Autodesk Inventor part; units mm, degrees
(part 3 of 3)
sketch "Эскиз6" plane through (0, 2, 0) normal (0, 1, 0) x (1, 0, 0)
  circle A0 centre (0, -40) radius 1.6 construction
  circle A1 centre (-46, 0) radius 1.6 construction
  circle A2 centre (46, 0) radius 1.6 construction
  line L0 (-6.2595, 46.1335) -> (-19.2746, 46.1335) construction
  arc A3 (-19.2746, 46.1335) -> (-21.6698, 47.1257) centre (-21.9203, 43.1335) ccw construction
  line L1 (-21.6698, 47.1257) -> (-42.4264, 67.8823) construction
  line L2 (-42.4264, 67.8823) -> (-34.2947, 76.014) construction
  arc A4 (-34.2947, 76.014) -> (-34.2947, 83.085) centre (-37.8302, 79.5495) ccw construction
  line L3 (-34.2947, 83.085) -> (-38.3892, 87.1795) construction
  arc A5 (-37.7453, 90.4395) -> (-38.3892, 87.1795) centre (-36.975, 88.5938) ccw construction
  arc A6 (-25.8102, 94.5401) -> (-37.7453, 90.4395) centre (0, 0) ccw construction
  arc A7 (-25.8102, 94.5401) -> (-20.7476, 95.7786) centre (-24, 98.1071) ccw construction
  arc A8 (20.7476, 95.7786) -> (-20.7476, 95.7786) centre (0, 0) ccw construction
  arc A9 (20.7476, 95.7786) -> (25.8102, 94.5401) centre (24, 98.1071) ccw construction
  arc A10 (37.7453, 90.4395) -> (25.8102, 94.5401) centre (0, 0) ccw construction
  arc A11 (38.3892, 87.1795) -> (37.7453, 90.4395) centre (36.975, 88.5938) ccw construction
  line L4 (38.3892, 87.1795) -> (34.2947, 83.085) construction
  arc A12 (34.2947, 83.085) -> (34.2947, 76.014) centre (37.8302, 79.5495) ccw construction
  line L5 (34.2947, 76.014) -> (42.4264, 67.8823) construction
  line L6 (42.4264, 67.8823) -> (21.6698, 47.1257) construction
  arc A13 (21.6698, 47.1257) -> (19.2746, 46.1335) centre (21.9203, 43.1335) ccw construction
  line L7 (19.2746, 46.1335) -> (6.2595, 46.1335) construction
  arc A14 (3.5768, 47.7906) -> (6.2595, 46.1335) centre (6.2595, 49.1335) ccw construction
  arc A15 (3.5768, 47.7906) -> (-3.5768, 47.7906) centre (0, 46) ccw construction
  arc A16 (-6.2595, 46.1335) -> (-3.5768, 47.7906) centre (-6.2595, 49.1335) ccw construction
  arc A17 (48.6481, 93.0503) -> (-48.6481, 93.0503) centre (0, 0) ccw construction
  arc A18 (-48.6481, 93.0503) -> (-49.3795, 88.2704) centre (-47.2582, 90.3917) ccw construction
  line L8 (-49.3795, 88.2704) -> (-46.3155, 85.2064) construction
  arc A19 (-46.3155, 73.8927) -> (-46.3155, 85.2064) centre (-51.9723, 79.5495) ccw construction
  line L9 (-46.3155, 73.8927) -> (-73.8927, 46.3155) construction
  arc A20 (-85.2064, 46.3155) -> (-73.8927, 46.3155) centre (-79.5495, 51.9723) ccw construction
  line L10 (-85.2064, 46.3155) -> (-88.2704, 49.3795) construction
  arc A21 (-88.2704, 49.3795) -> (-93.0503, 48.6481) centre (-90.3917, 47.2582) ccw construction
  arc A22 (-93.0503, 48.6481) -> (-93.0503, -48.6481) centre (0, 0) ccw construction
  arc A23 (-93.0503, -48.6481) -> (-88.2704, -49.3795) centre (-90.3917, -47.2582) ccw construction
  line L11 (-88.2704, -49.3795) -> (-85.2064, -46.3155) construction
  arc A24 (-73.8927, -46.3155) -> (-85.2064, -46.3155) centre (-79.5495, -51.9723) ccw construction
  line L12 (-73.8927, -46.3155) -> (-46.3155, -73.8927) construction
  arc A25 (-46.3155, -85.2064) -> (-46.3155, -73.8927) centre (-51.9723, -79.5495) ccw construction
  line L13 (-46.3155, -85.2064) -> (-49.3795, -88.2704) construction
  arc A26 (-49.3795, -88.2704) -> (-48.6481, -93.0503) centre (-47.2582, -90.3917) ccw construction
  arc A27 (-48.6481, -93.0503) -> (-45.42, -94.668) centre (0, 0) ccw construction
  arc A28 (-45.42, -94.668) -> (-43.0355, -94.1655) centre (-44.5548, -92.8648) ccw construction
  line L14 (-43.0355, -94.1655) -> (-18.3802, -65.3664) construction
  arc A29 (-17.477, -64.7643) -> (-18.3802, -65.3664) centre (-16.8609, -66.6671) ccw construction
  line L15 (-17.477, -64.7643) -> (-0.6161, -59.3045) construction
  arc A30 (0.6161, -59.3045) -> (-0.6161, -59.3045) centre (0, -61.2072) ccw construction
  line L16 (0.6161, -59.3045) -> (17.477, -64.7643) construction
  arc A31 (18.3802, -65.3664) -> (17.477, -64.7643) centre (16.8609, -66.6671) ccw construction
  line L17 (18.3802, -65.3664) -> (43.0355, -94.1655) construction
  arc A32 (43.0355, -94.1655) -> (45.42, -94.668) centre (44.5548, -92.8648) ccw construction
  arc A33 (45.42, -94.668) -> (48.6481, -93.0503) centre (0, 0) ccw construction
  arc A34 (48.6481, -93.0503) -> (49.3795, -88.2704) centre (47.2582, -90.3917) ccw construction
  line L18 (49.3795, -88.2704) -> (46.3155, -85.2064) construction
  arc A35 (46.3155, -73.8927) -> (46.3155, -85.2064) centre (51.9723, -79.5495) ccw construction
  line L19 (46.3155, -73.8927) -> (73.8927, -46.3155) construction
  arc A36 (85.2064, -46.3155) -> (73.8927, -46.3155) centre (79.5495, -51.9723) ccw construction
  line L20 (85.2064, -46.3155) -> (88.2704, -49.3795) construction
  arc A37 (88.2704, -49.3795) -> (93.0503, -48.6481) centre (90.3917, -47.2582) ccw construction
  arc A38 (93.0503, -48.6481) -> (93.0503, 48.6481) centre (0, 0) ccw construction
  arc A39 (93.0503, 48.6481) -> (88.2704, 49.3795) centre (90.3917, 47.2582) ccw construction
  line L21 (88.2704, 49.3795) -> (85.2064, 46.3155) construction
  arc A40 (73.8927, 46.3155) -> (85.2064, 46.3155) centre (79.5495, 51.9723) ccw construction
  line L22 (73.8927, 46.3155) -> (46.3155, 73.8927) construction
  arc A41 (46.3155, 85.2064) -> (46.3155, 73.8927) centre (51.9723, 79.5495) ccw construction
  line L23 (46.3155, 85.2064) -> (49.3795, 88.2704) construction
  arc A42 (49.3795, 88.2704) -> (48.6481, 93.0503) centre (47.2582, 90.3917) ccw construction
  circle A43 centre (-24, 98.1071) radius 1.6 construction
  arc A44 (47.7906, -3.5768) -> (46.1335, -6.2595) centre (49.1335, -6.2595) ccw construction
  arc A45 (47.7906, -3.5768) -> (47.7906, 3.5768) centre (46, 0) ccw construction
  arc A46 (46.1335, 6.2595) -> (47.7906, 3.5768) centre (49.1335, 6.2595) ccw construction
  line L24 (46.1335, 6.2595) -> (46.1335, 19.2746) construction
  arc A47 (46.1335, 19.2746) -> (47.1257, 21.6698) centre (43.1335, 21.9203) ccw construction
  line L25 (47.1257, 21.6698) -> (67.8823, 42.4264) construction
  line L26 (67.8823, 42.4264) -> (76.014, 34.2947) construction
  arc A48 (76.014, 34.2947) -> (83.085, 34.2947) centre (79.5495, 37.8302) ccw construction
  line L27 (83.085, 34.2947) -> (87.1795, 38.3892) construction
  arc A49 (90.4395, 37.7453) -> (87.1795, 38.3892) centre (88.5938, 36.975) ccw construction
  arc A50 (97.9653, 2.6059) -> (90.4395, 37.7453) centre (0, 0) ccw construction
  arc A51 (97.9653, 2.6059) -> (97.9653, -2.6059) centre (101, 0) ccw construction
  arc A52 (90.4395, -37.7453) -> (97.9653, -2.6059) centre (0, 0) ccw construction
  arc A53 (87.1795, -38.3892) -> (90.4395, -37.7453) centre (88.5938, -36.975) ccw construction
  line L28 (87.1795, -38.3892) -> (83.085, -34.2947) construction
  arc A54 (83.085, -34.2947) -> (76.014, -34.2947) centre (79.5495, -37.8302) ccw construction
  line L29 (76.014, -34.2947) -> (67.8823, -42.4264) construction
  line L30 (67.8823, -42.4264) -> (47.1257, -21.6698) construction
  arc A55 (47.1257, -21.6698) -> (46.1335, -19.2746) centre (43.1335, -21.9203) ccw construction
  line L31 (46.1335, -19.2746) -> (46.1335, -6.2595) construction
  circle A56 centre (101, 0) radius 1.6 construction
  circle A57 centre (-101, 0) radius 1.6 construction
  arc A58 (-47.7906, 3.5768) -> (-46.1335, 6.2595) centre (-49.1335, 6.2595) ccw construction
  arc A59 (-47.7906, 3.5768) -> (-47.7906, -3.5768) centre (-46, 0) ccw construction
  arc A60 (-46.1335, -6.2595) -> (-47.7906, -3.5768) centre (-49.1335, -6.2595) ccw construction
  line L32 (-46.1335, -6.2595) -> (-46.1335, -19.2746) construction
  arc A61 (-46.1335, -19.2746) -> (-47.1257, -21.6698) centre (-43.1335, -21.9203) ccw construction
  line L33 (-47.1257, -21.6698) -> (-67.8823, -42.4264) construction
  line L34 (-67.8823, -42.4264) -> (-76.014, -34.2947) construction
  arc A62 (-76.014, -34.2947) -> (-83.085, -34.2947) centre (-79.5495, -37.8302) ccw construction
  line L35 (-83.085, -34.2947) -> (-87.1795, -38.3892) construction
  arc A63 (-90.4395, -37.7453) -> (-87.1795, -38.3892) centre (-88.5938, -36.975) ccw construction
  arc A64 (-97.9653, -2.6059) -> (-90.4395, -37.7453) centre (0, 0) ccw construction
  arc A65 (-97.9653, -2.6059) -> (-97.9653, 2.6059) centre (-101, 0) ccw construction
  arc A66 (-90.4395, 37.7453) -> (-97.9653, 2.6059) centre (0, 0) ccw construction
  arc A67 (-87.1795, 38.3892) -> (-90.4395, 37.7453) centre (-88.5938, 36.975) ccw construction
  line L36 (-87.1795, 38.3892) -> (-83.085, 34.2947) construction
  arc A68 (-83.085, 34.2947) -> (-76.014, 34.2947) centre (-79.5495, 37.8302) ccw construction
  line L37 (-76.014, 34.2947) -> (-67.8823, 42.4264) construction
  line L38 (-67.8823, 42.4264) -> (-47.1257, 21.6698) construction
  arc A69 (-47.1257, 21.6698) -> (-46.1335, 19.2746) centre (-43.1335, 21.9203) ccw construction
  line L39 (-46.1335, 19.2746) -> (-46.1335, 6.2595) construction
  circle A70 centre (45.1111, -90.3659) radius 1.6 construction
  circle A71 centre (45.1111, 90.3659) radius 1.6 construction
  circle A72 centre (90.3659, 45.1111) radius 1.6 construction
  circle A73 centre (-45.1111, -90.3659) radius 1.6 construction
  circle A74 centre (90.3659, -45.1111) radius 1.6 construction
  circle A75 centre (-45.1111, 90.3659) radius 1.6 construction
  circle A76 centre (-90.3659, 45.1111) radius 1.6 construction
  circle A77 centre (-90.3659, -45.1111) radius 1.6 construction
  line L40 (63.6396, 46.669) -> (43.8406, 26.8701) construction
  arc A78 (41.0122, 26.8701) -> (43.8406, 26.8701) centre (42.4264, 28.2843) ccw construction
  line L41 (41.0122, 26.8701) -> (26.8701, 41.0122) construction
  arc A79 (26.8701, 43.8406) -> (26.8701, 41.0122) centre (28.2843, 42.4264) ccw construction
  line L42 (26.8701, 43.8406) -> (46.669, 63.6396) construction
  line L43 (46.669, 63.6396) -> (63.6396, 46.669) construction
  line L44 (-46.669, 63.6396) -> (-26.8701, 43.8406) construction
  arc A80 (-26.8701, 41.0122) -> (-26.8701, 43.8406) centre (-28.2843, 42.4264) ccw construction
  line L45 (-26.8701, 41.0122) -> (-41.0122, 26.8701) construction
  arc A81 (-43.8406, 26.8701) -> (-41.0122, 26.8701) centre (-42.4264, 28.2843) ccw construction
  line L46 (-43.8406, 26.8701) -> (-63.6396, 46.669) construction
  line L47 (-63.6396, 46.669) -> (-46.669, 63.6396) construction
  line L48 (-63.6396, -46.669) -> (-43.8406, -26.8701) construction
  arc A82 (-41.0122, -26.8701) -> (-43.8406, -26.8701) centre (-42.4264, -28.2843) ccw construction
  line L49 (-41.0122, -26.8701) -> (-26.8701, -41.0122) construction
  arc A83 (-26.8701, -43.8406) -> (-26.8701, -41.0122) centre (-28.2843, -42.4264) ccw construction
  line L50 (-26.8701, -43.8406) -> (-46.669, -63.6396) construction
  line L51 (-46.669, -63.6396) -> (-63.6396, -46.669) construction
  line L52 (-42.4264, -67.8823) -> (-21.6698, -47.1257) construction
  arc A84 (-21.6698, -47.1257) -> (-19.2746, -46.1335) centre (-21.9203, -43.1335) ccw construction
  line L53 (-19.2746, -46.1335) -> (19.2746, -46.1335) construction
  arc A85 (19.2746, -46.1335) -> (21.6698, -47.1257) centre (21.9203, -43.1335) ccw construction
  line L54 (21.6698, -47.1257) -> (42.4264, -67.8823) construction
  line L55 (42.4264, -67.8823) -> (37.1244, -73.1843) construction
  arc A86 (34.1909, -73.0707) -> (37.1244, -73.1843) centre (35.7102, -71.7701) ccw construction
  line L56 (34.1909, -73.0707) -> (25.4187, -62.8242) construction
  arc A87 (24.842, -61.8893) -> (25.4187, -62.8242) centre (28.1154, -60.5155) ccw construction
  line L57 (24.842, -61.8893) -> (23.8313, -59.4808) construction
  arc A88 (23.8313, -59.4808) -> (21.0049, -57.3328) centre (20.5578, -60.8546) ccw construction
  line L58 (21.0049, -57.3328) -> (15.1585, -56.5907) construction
  arc A89 (14.5119, -56.4463) -> (15.1585, -56.5907) centre (15.6055, -53.069) ccw construction
  line L59 (14.5119, -56.4463) -> (0.6161, -51.9466) construction
  arc A90 (0.6161, -51.9466) -> (-0.6161, -51.9466) centre (0, -53.8493) ccw construction
  line L60 (-0.6161, -51.9466) -> (-14.5119, -56.4463) construction
  arc A91 (-15.1585, -56.5907) -> (-14.5119, -56.4463) centre (-15.6055, -53.069) ccw construction
  line L61 (-15.1585, -56.5907) -> (-21.0049, -57.3328) construction
  arc A92 (-21.0049, -57.3328) -> (-23.8313, -59.4808) centre (-20.5578, -60.8546) ccw construction
  line L62 (-23.8313, -59.4808) -> (-24.842, -61.8893) construction
  arc A93 (-25.4187, -62.8242) -> (-24.842, -61.8893) centre (-28.1154, -60.5155) ccw construction
  line L63 (-25.4187, -62.8242) -> (-34.1909, -73.0707) construction
  arc A94 (-37.1244, -73.1843) -> (-34.1909, -73.0707) centre (-35.7102, -71.7701) ccw construction
  line L64 (-37.1244, -73.1843) -> (-42.4264, -67.8823) construction
  circle A95 centre (43.1335, 21.9203) radius 1.6 construction
  circle A96 centre (21.9203, -43.1335) radius 1.6 construction
  circle A97 centre (-21.9203, -43.1335) radius 1.6 construction
  circle A98 centre (-43.1335, -21.9203) radius 1.6 construction
  circle A99 centre (-43.1335, 21.9203) radius 1.6 construction
  circle A100 centre (-21.9203, 43.1335) radius 1.6 construction
  circle A101 centre (43.1335, -21.9203) radius 1.6 construction
  circle A102 centre (21.9203, 43.1335) radius 1.6 construction
  circle A103 centre (-37.8302, 79.5495) radius 1.6 construction
  circle A104 centre (-79.5495, 37.8302) radius 1.6 construction
  circle A105 centre (-79.5495, -37.8302) radius 1.6 construction
  circle A106 centre (79.5495, -37.8302) radius 1.6 construction
  circle A107 centre (37.8302, 79.5495) radius 1.6 construction
  circle A108 centre (79.5495, 37.8302) radius 1.6 construction
  circle A109 centre (-20.5578, -60.8546) radius 1.55 construction
  circle A110 centre (20.5578, -60.8546) radius 1.55 construction
  circle A111 centre (37.8302, -79.5495) radius 1.6 construction
  circle A112 centre (-37.8302, -79.5495) radius 1.6 construction
  line L65 (46.669, -63.6396) -> (26.8701, -43.8406) construction
  arc A113 (26.8701, -41.0122) -> (26.8701, -43.8406) centre (28.2843, -42.4264) ccw construction
  line L66 (26.8701, -41.0122) -> (41.0122, -26.8701) construction
  arc A114 (43.8406, -26.8701) -> (41.0122, -26.8701) centre (42.4264, -28.2843) ccw construction
  line L67 (43.8406, -26.8701) -> (63.6396, -46.669) construction
  line L68 (63.6396, -46.669) -> (46.669, -63.6396) construction
  circle A115 centre (24, 98.1071) radius 1.6 construction
  circle A116 centre (0, 46) radius 1.6 construction
  arc A117 (3.6492, -38.362) -> (6.3862, -40.1335) centre (6.3862, -37.1335) ccw construction
  arc A118 (3.6492, -38.362) -> (-3.6492, -38.362) centre (0, -40) ccw construction
  arc A119 (-6.3862, -40.1335) -> (-3.6492, -38.362) centre (-6.3862, -37.1335) ccw construction
  line L69 (-6.3862, -40.1335) -> (-19.2746, -40.1335) construction
  arc A120 (-19.2746, -40.1335) -> (-21.6698, -39.1414) centre (-21.9203, -43.1335) ccw construction
  line L70 (-21.6698, -39.1414) -> (-39.1414, -21.6698) construction
  arc A121 (-39.1414, -21.6698) -> (-40.1335, -19.2746) centre (-43.1335, -21.9203) ccw construction
  line L71 (-40.1335, -19.2746) -> (-40.1335, 19.2746) construction
  arc A122 (-40.1335, 19.2746) -> (-39.1414, 21.6698) centre (-43.1335, 21.9203) ccw construction
  line L72 (-39.1414, 21.6698) -> (-21.6698, 39.1414) construction
  arc A123 (-21.6698, 39.1414) -> (-19.2746, 40.1335) centre (-21.9203, 43.1335) ccw construction
  line L73 (-19.2746, 40.1335) -> (19.2746, 40.1335) construction
  arc A124 (19.2746, 40.1335) -> (21.6698, 39.1414) centre (21.9203, 43.1335) ccw construction
  line L74 (21.6698, 39.1414) -> (39.1414, 21.6698) construction
  arc A125 (39.1414, 21.6698) -> (40.1335, 19.2746) centre (43.1335, 21.9203) ccw construction
  line L75 (40.1335, 19.2746) -> (40.1335, -19.2746) construction
  arc A126 (40.1335, -19.2746) -> (39.1414, -21.6698) centre (43.1335, -21.9203) ccw construction
  line L76 (39.1414, -21.6698) -> (21.6698, -39.1414) construction
  arc A127 (21.6698, -39.1414) -> (19.2746, -40.1335) centre (21.9203, -43.1335) ccw construction
  line L77 (19.2746, -40.1335) -> (6.3862, -40.1335) construction
  line L78 (0, 0) -> (0, 105) construction
  arc A128 (48.6481, 93.0503) -> (-48.6481, 93.0503) centre (0, 0) ccw construction
  line L79 (-19.5, 5.5231) -> (19.5, 5.5231) construction
  line L80 (19.5, 5.5231) -> (19.5, 136.6901) construction
  line L81 (19.5, 136.6901) -> (-19.5, 136.6901) construction
  line L82 (-19.5, 136.6901) -> (-19.5, 5.5231) construction
  circle A129 centre (-24, 98.1071) radius 4 construction
  circle A130 centre (24, 98.1071) radius 4 construction
  arc A131 (-21.3158, 95.1414) -> (20.4598, 95.3292) centre (0, 0) ccw construction
  arc A132 (-23.5, 93.6349) -> (-20.4598, 95.3292) centre (-24, 98.1071) ccw
  line L83 (-23.5, 49.663) -> (-23.5, 93.6349)
  line L84 (-20, 47.2032) -> (-20, 95.4267)
  arc A133 (-19.0919, 46.6335) -> (-21.4454, 47.6084) centre (-21.9203, 43.1335) ccw
  line L85 (-21.4454, 47.6084) -> (-23.5, 49.663)
  line L86 (-21.6698, 47.1257) -> (-42.4264, 67.8823) construction
  line L87 (-42.4264, 67.8823) -> (-34.2947, 76.014) construction
  line L88 (-19.0919, 46.6335) -> (-6.5611, 46.6335)
  arc A134 (0, 41.5) -> (3.9366, 48.1801) centre (0, 46) ccw construction
  arc A135 (-4.4552, 46.6335) -> (0, 41.5) centre (0, 46) ccw construction
  arc A136 (-6.5611, 46.6335) -> (-3.9366, 48.1801) centre (-6.5611, 49.6335) ccw
  line L89 (-23.5, 49.663) -> (-42.0729, 68.2358) construction
  arc A137 (-18.5662, 46.1335) -> (-19.0919, 46.6335) centre (-21.9203, 43.1335) ccw construction
  arc A138 (-21.4454, 47.6084) -> (-18.5662, 46.1335) centre (-21.9203, 43.1335) ccw construction
  arc A139 (-25.858, 94.0086) -> (-23.5, 93.6349) centre (-24, 98.1071) ccw construction
  arc A140 (-20.4598, 95.3292) -> (-25.858, 94.0086) centre (-24, 98.1071) ccw construction
  arc A141 (-20.4598, 95.3292) -> (-21.3158, 95.1414) centre (0, 0) ccw construction
  arc A142 (20.4598, 95.3292) -> (23.5, 93.6349) centre (24, 98.1071) ccw
  line L90 (23.5, 49.663) -> (23.5, 93.6349)
  line L91 (20, 47.2032) -> (20, 95.4267)
  arc A143 (21.4454, 47.6084) -> (19.0919, 46.6335) centre (21.9203, 43.1335) ccw
  line L92 (21.4454, 47.6084) -> (23.5, 49.663)
  line L93 (19.0919, 46.6335) -> (6.5611, 46.6335)
  arc A144 (3.9366, 48.1801) -> (6.5611, 46.6335) centre (6.5611, 49.6335) ccw
  arc A145 (3.9366, 48.1801) -> (-3.9366, 48.1801) centre (0, 46) ccw
  arc A146 (20.4598, 95.3292) -> (-20.4598, 95.3292) centre (0, 0) ccw
  dimension "d26" = 360
  dimension "d112" = 8
  dimension "d111" = 39
  dimension "d113" = 0.5
  dimension "d114" = 9
  dimension "d115" = 4
  dimension "d116" = 0.5
  dimension "d117" = 9
  dimension "d118" = 0.5
  dimension "d119" = 0.5
  dimension "d120" = 9
  dimension "d121" = 3
  constraints: 42 point on circle, 28 end point, 17 centre point, 13 symmetric about line, 5 coincident, 4 parallel, 4 point on line, 2 horizontal, 2 tangent, 2 vertical, 1 perpendicular, 8 other
  measures "d111" distance of L81.end L80.end
  measures "d113" radial gap between concentric circles of A8 A131
  measures "d114" diameter of A132
  measures "d115" distance between parallel lines of L82 L83
  measures "d116" distance between parallel lines of L82 L84
  measures "d117" diameter of A133
  measures "d118" distance between parallel lines of L86 L85
  measures "d119" distance between parallel lines of L0 L88
  measures "d120" diameter of A134
  measures "d121" radius of A136
extrude "Выдавливание9" add sketch "Эскиз6" along normal blind 1.85 and the other way blind 2
extrude "Выдавливание10" add sketch "Эскиз6" along normal blind 7 contours A132 A146 L84 A133 L85 L83 | A146 A142 L90 L92 A143 L91
ref_plane "РабПлоскость1" through (0, 9, 0) normal (0, 1, 0) x (1, 0, 0)
sketch "Эскиз7" plane through (0, 9, 0) normal (0, 1, 0) x (1, 0, 0)
  line L0 (-20, 95.4267) -> (-20, 47.2032) projected
  arc A0 (-19.0919, 46.6335) -> (-20, 47.2032) centre (-21.9203, 43.1335) ccw projected
  line L1 (-19.0919, 46.6335) -> (-6.5611, 46.6335) projected
  arc A1 (-6.5611, 46.6335) -> (-3.9366, 48.1801) centre (-6.5611, 49.6335) ccw construction
  arc A2 (3.9366, 48.1801) -> (-3.9366, 48.1801) centre (0, 46) ccw construction
  arc A3 (3.9366, 48.1801) -> (6.5611, 46.6335) centre (6.5611, 49.6335) ccw construction
  line L2 (6.5611, 46.6335) -> (19.0919, 46.6335) projected
  arc A4 (20, 47.2032) -> (19.0919, 46.6335) centre (21.9203, 43.1335) ccw projected
  line L3 (20, 47.2032) -> (20, 95.4267) projected
  arc A5 (20, 95.4267) -> (-20, 95.4267) centre (0, 0) ccw projected
  arc A6 (-20, 95.4267) -> (-20.4598, 95.3292) centre (0, 0) ccw projected
  arc A7 (-23.5, 93.6349) -> (-20.4598, 95.3292) centre (-24, 98.1071) ccw projected
  line L4 (-23.5, 93.6349) -> (-23.5, 49.663) projected
  line L5 (-23.5, 49.663) -> (-21.4454, 47.6084) projected
  arc A8 (-20, 47.2032) -> (-21.4454, 47.6084) centre (-21.9203, 43.1335) ccw projected
  line L6 (-20, 47.2032) -> (-20, 95.4267) projected
  arc A9 (20.4598, 95.3292) -> (20, 95.4267) centre (0, 0) ccw projected
  line L7 (20, 95.4267) -> (20, 47.2032) projected
  arc A10 (21.4454, 47.6084) -> (20, 47.2032) centre (21.9203, 43.1335) ccw projected
  line L8 (21.4454, 47.6084) -> (23.5, 49.663) projected
  line L9 (23.5, 49.663) -> (23.5, 93.6349) projected
  arc A11 (20.4598, 95.3292) -> (23.5, 93.6349) centre (24, 98.1071) ccw projected
  line L10 (18.2, 46.6335) -> (18.2, 95.7863)
  arc A12 (3.5768, 47.7906) -> (-3.5768, 47.7906) centre (0, 46) ccw construction
  line L11 (0, 46) -> (0, 97.5) construction
  line L12 (-18.2, 46.6335) -> (-18.2, 95.7863)
  point P0 (-20, 95.4267)
  point P1 (20, 95.4267)
  dimension "d129" = 1.8
  constraints: 6 end point, 2 point on circle, 2 symmetric about line, 1 point on line, 1 vertical
  measures "d129" distance between parallel lines of L3 L10
extrude "Выдавливание11" add sketch "Эскиз7" along normal blind 5
chamfer "Фаска1" distance 1.8 angle 45 2 edges at (18.2, 9, -71.2099) (-18.2, 9, -71.2099)
fillet "Сопряжение1" radius 3 2 edges at (23.5, 14, -71.6489) (-23.5, 14, -71.6489)
fillet "Сопряжение2" radius 1 2 edges at (18.2, 14, -71.2099) (-18.2, 14, -71.2099)
ref_plane "РабПлоскость2" through (6.5611, 3.85, -46.6335) normal (0, 0, 1) x (1, 0, 0)
sketch "Эскиз8" plane through (6.5611, 3.85, -46.6335) normal (0, 0, 1) x (1, 0, 0)
  line L0 (-26.5611, 0) -> (-25.6529, 0) construction
  line L1 (-25.6529, 0) -> (-13.1221, 0) construction
  line L2 (-13.1221, 0) -> (-10.4977, 0) construction
  line L3 (-10.4977, 0) -> (-2.6244, 0) construction
  line L4 (-2.6244, 0) -> (0, 0) construction
  line L5 (0, 0) -> (12.5308, 0) construction
  line L6 (12.5308, 0) -> (13.4389, 0) construction
  line L7 (13.4389, 0) -> (-26.5611, 0) construction
  line L8 (-24.7611, 6.95) -> (-24.7611, 9.15) construction
  line L9 (-26.5611, 5.15) -> (-24.7611, 6.95) construction
  line L10 (-26.5611, 0) -> (-26.5611, 5.15) construction
  line L11 (13.4389, 0) -> (-26.5611, 0) construction
  line L12 (13.4389, 0) -> (13.4389, 5.15) construction
  line L13 (11.6389, 6.95) -> (13.4389, 5.15) construction
  line L14 (11.6389, 6.95) -> (11.6389, 9.15) construction
  line L15 (13.8987, 10.15) -> (12.6389, 10.15) construction
  line L16 (13.8987, -3.85) -> (13.8987, 10.15) construction
  line L17 (-27.0209, -3.85) -> (13.8987, -3.85) construction
  line L18 (-27.0209, -3.85) -> (-27.0209, 10.15) construction
  line L19 (-25.7611, 10.15) -> (-27.0209, 10.15) construction
  line L20 (-27.0209, 10.15) -> (-27.0611, 10.15) construction
  line L21 (-27.0209, -3.85) -> (-27.0209, 10.15) construction
  line L22 (-30.0611, -3.85) -> (-27.0209, -3.85) construction
  line L23 (-30.0611, -3.85) -> (-30.0611, 7.15) construction
  line L24 (16.9389, -3.85) -> (16.9389, 7.15) construction
  line L25 (13.8987, -3.85) -> (16.9389, -3.85) construction
  line L26 (13.8987, -3.85) -> (13.8987, 10.15) construction
  line L27 (13.9389, 10.15) -> (13.8987, 10.15) construction
  line L28 (-6.5611, -3.85) -> (-6.5611, 0) construction
  line L29 (-6.5611, -1.85) -> (-6.5611, 0.15) construction
  line L30 (-8.1611, -1.85) -> (-4.9611, -1.85) construction
  line L31 (-11.4446, 0.15) -> (-1.6776, 0.15) construction
  line L32 (-6.5611, -1.85) -> (-4.0611, -1.85) construction
  line L33 (-4.0611, -1.85) -> (-1.6776, 0.15) construction
  line L34 (-6.5611, -1.85) -> (-9.0611, -1.85) construction
  line L35 (-9.0611, -1.85) -> (-11.4446, 0.15) construction
  line L36 (-11.7325, 0) -> (-9.5278, -1.85)
  line L37 (-2.9842, -1.85) -> (-10.1379, -1.85) construction
  line L38 (-1.3896, 0) -> (-3.5943, -1.85)
  line L39 (-1.3896, 0) -> (-11.7325, 0)
  line L40 (13.4389, 0) -> (-26.5611, 0) projected
  line L41 (-9.5278, -1.85) -> (-3.5943, -1.85)
  dimension "d138" = 2
  dimension "d139" = 2.5
  dimension "d141" = 40
  dimension "d142" = 0.3
  constraints: 22 end point, 5 point on line, 4 symmetric about line, 3 midpoint, 2 collinear, 2 parallel, 1 horizontal, 5 other
  measures "d138" distance of L29.start L29.end
  measures "d139" distance of L29.start L32.end
  measures "d141" angle of L31 L33
  measures "d142" distance between parallel lines of L35 L36
extrude "Выдавливание12" cut sketch "Эскиз8" against normal mid plane 300
